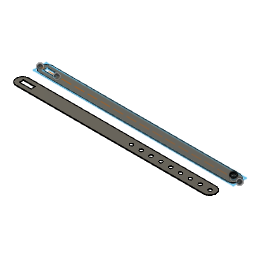
prusa-shield-headband v2 (Autodesk Fusion 360 design; units mm, degrees)
Autodesk Fusion 360 part; units mm, degrees
sketch "Sketch1" plane through (0, 0, 0) normal (0, 0, 1) x (1, 0, 0) in component "headband"
  line L0 (12.1287, -0.0199) -> (215.3287, -0.0199)
  line L1 (215.3287, -0.0199) -> (215.3287, 12.6801)
  line L2 (215.3287, 12.6801) -> (12.1287, 12.6801)
  line L3 (12.1287, 12.6801) -> (12.1287, -0.0199)
  line L4 (17.1287, 8.4301) -> (29.1287, 8.4301)
  line L5 (29.1287, 8.4301) -> (29.1287, 4.2301)
  line L6 (29.1287, 4.2301) -> (17.1287, 4.2301)
  line L7 (17.1287, 4.2301) -> (17.1287, 8.4301)
  line L8 (215.3287, 6.3301) -> (12.1287, 6.3301) construction
  circle A0 centre (209.3287, 6.3301) radius 1.5
  point P0 (12.1287, 6.3301)
  point P1 (215.3287, 6.3301)
  point P2 (29.1287, 6.3301)
  dimension "d1" = 12.7
  dimension "d2" = 12
  dimension "d3" = 4.2
  dimension "d4" = 203.2
  dimension "d5" = 5
  dimension "d6" = 3
  dimension "d20" = 6
  constraint horizontal L0
  constraint vertical L1
  constraint horizontal L2
  constraint vertical L3
  constraint horizontal L4
  constraint vertical L5
  constraint horizontal L6
  constraint vertical L7
  constraint midpoint L3 P0
  constraint midpoint L1 P1
  constraint coincident P1 L8.start
  constraint coincident P0 L8.end
  constraint midpoint L5 P2
  constraint coincident L8 P2
  constraint coincident L8 A0.centre
  measures "d1" distance of L0.start L2.end
  measures "d2" distance of L4.start L4.end
  measures "d3" distance of L4.end L5.end
  measures "d4" distance of L1.end L2.end
  measures "d5" distance of L3 L4.start
  measures "d6" diameter of A0
  measures "d20" distance of L1 A0.centre
extrude "Extrude1" add sketch "Sketch1" along normal blind 0.6 contours L0 L1 L2 L3 | A0 makes body 1 in component "headband"
fillet "Fillet1" radius 6 1 edges at (215.3287, -0.0199, 0.3) on bodies 1 in component "headband"
fillet "Fillet2" radius 6 1 edges at (215.3287, 12.6801, 0.3) on bodies 1 in component "headband"
fillet "Fillet3" radius 6 1 edges at (12.1287, 12.6801, 0.3) on bodies 1 in component "headband"
fillet "Fillet4" radius 6 1 edges at (12.1287, -0.0199, 0.3) on bodies 1 in component "headband"
extrude "Extrude2" add sketch "Sketch1" along normal blind 3 contours A0 bodies 1 in component "headband"
sketch "Sketch2" plane through (0, 0, 3) normal (0, 0, 1) x (-1, 0, 0) in component "headband"
  circle A0 centre (-209.3287, -6.3301) radius 1.5
  circle A1 centre (-209.3287, -6.3301) radius 2.5
  dimension "d15" = 5
  constraint concentric A0 A1
  measures "d15" diameter of A1
extrude "Extrude3" add sketch "Sketch2" along normal blind 1 contours A0 | A1 bodies 1 in component "headband"
sketch "Sketch3" plane through (0, 0, 0) normal (1, 0, 0) x (0, 1, 0) in component "headband"
fillet "Fillet5" radius 1.25 1 edges at (207.9302, 5.7877, 3) on bodies 1 in component "headband"
fillet "Fillet6" radius 1 1 edges at (211.6595, 7.2341, 4) on bodies 1 in component "headband"
sketch "Sketch1 (2)" plane through (0, 0, 0) normal (0, 0, 1) x (1, 0, 0) in component "receiverband"
  line L0 (10.8146, -10.1244) -> (214.0146, -10.1244)
  line L1 (214.0146, -10.1244) -> (214.0146, -22.8244)
  line L2 (214.0146, -22.8244) -> (10.8146, -22.8244)
  line L3 (10.8146, -22.8244) -> (10.8146, -10.1244)
  line L4 (15.8146, -14.3744) -> (27.8146, -14.3744)
  line L5 (27.8146, -14.3744) -> (27.8146, -18.5744)
  line L6 (27.8146, -18.5744) -> (15.8146, -18.5744)
  line L7 (15.8146, -18.5744) -> (15.8146, -14.3744)
  line L8 (214.0146, -16.4744) -> (10.8146, -16.4744) construction
  circle A0 centre (208.0146, -16.4744) radius 1.7
  circle A1 centre (198.0146, -16.4744) radius 1.7
  circle A2 centre (188.0146, -16.4744) radius 1.7
  circle A3 centre (178.0146, -16.4744) radius 1.7
  circle A4 centre (168.0146, -16.4744) radius 1.7
  circle A5 centre (158.0146, -16.4744) radius 1.7
  circle A6 centre (148.0146, -16.4744) radius 1.7
  circle A7 centre (138.0146, -16.4744) radius 1.7
  circle A8 centre (128.0146, -16.4744) radius 1.7
  point P0 (10.8146, -16.4744)
  point P1 (214.0146, -16.4744)
  point P2 (27.8146, -16.4744)
  point P3 (128.0146, -16.4744)
  dimension "d23" = 12.7
  dimension "d24" = 203.2
  dimension "d25" = 4.2
  dimension "d26" = 12
  dimension "d27" = 5
  dimension "d28" = 3.4
  dimension "d29" = 6
  dimension "d30" = 3.4
  dimension "d31" = 3.4
  dimension "d32" = 3.4
  dimension "d33" = 10
  dimension "d34" = 10
  dimension "d35" = 10
  dimension "d43" = 3.4
  dimension "d44" = 3.4
  dimension "d45" = 10
  dimension "d46" = 10
  dimension "d47" = 3.4
  dimension "d48" = 3.4
  dimension "d49" = 3.4
  constraint horizontal L0
  constraint vertical L1
  constraint horizontal L2
  constraint vertical L3
  constraint horizontal L4
  constraint vertical L5
  constraint horizontal L6
  constraint vertical L7
  constraint midpoint L3 P0
  constraint midpoint L1 P1
  constraint coincident P1 L8.start
  constraint coincident P0 L8.end
  constraint midpoint L5 P2
  constraint coincident L8 P2
  constraint coincident L8 A0.centre
  constraint coincident L8 A1.centre
  constraint coincident L8 A2.centre
  constraint coincident L8 A3.centre
  constraint coincident L8 A4.centre
  constraint coincident L8 A5.centre
  measures "d23" distance of L0.start L2.end
  measures "d24" distance of L1.end L2.end
  measures "d25" distance of L4.end L5.end
  measures "d26" distance of L4.start L4.end
  measures "d27" distance of L3 L7
  measures "d28" diameter of A0
  measures "d29" distance of P1 A0.centre
  measures "d30" diameter of A1
  measures "d31" diameter of A2
  measures "d32" diameter of A3
  measures "d33" distance of A0.centre A1.centre
  measures "d34" distance of A1.centre A2.centre
  measures "d35" distance of A2.centre A3.centre
  measures "d43" diameter of A4
  measures "d44" diameter of A5
  measures "d45" distance of A3.centre A4.centre
  measures "d46" distance of A4.centre A5.centre
  measures "d47" diameter of A6
  measures "d48" diameter of A7
  measures "d49" diameter of A8
extrude "Extrude1'" add sketch "Sketch1 (2)" along normal blind 0.6 separate body makes body 2 in component "receiverband"
fillet "Fillet1'" radius 6 2 edges at (10.8146, -22.8244, 0.3) (10.8146, -10.1244, 0.3) on bodies 2 in component "receiverband"
fillet "Fillet2'" radius 6 2 edges at (214.0146, -10.1244, 0.3) (214.0146, -22.8244, 0.3) on bodies 2 in component "receiverband"
component "headband" placed x (1, 0, 0) y (0, 1, 0) z (0, 0, 1) at (0, 0, 0)
component "receiverband" placed x (1, 0, 0) y (0, 1, 0) z (0, 0, 1) at (0, 0, 0)
equation "d1 = bandwidth"
equation "d2 = slotlength"
equation "d3 = slotwidth"
equation "d4 = bandlength"
equation "d7 = bandthick"
equation "bandlength = 8 in"
equation "bandwidth = 0.5 in"
equation "d23 = bandwidth"
equation "d24 = bandlength"
equation "d25 = slotwidth"
equation "d26 = slotlength"
equation "d30 = d28"
equation "d31 = d28"
equation "d32 = d28"
equation "d36 = bandthick"
equation "bandthick = 0.6 mm"
equation "slotlength = 12 mm"
equation "slotwidth = 4.2 mm"
equation "d43 = d28"
equation "d44 = d28"
equation "d47 = d28"
equation "d48 = d28"
equation "d49 = d28"
